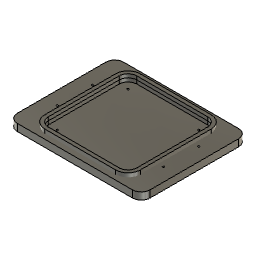
actu_board v5 (Autodesk Fusion 360 design; units mm, degrees)
Autodesk Fusion 360 part; units mm, degrees
sketch "스케치1" plane through (0, 0, 0) normal (0, 0, 1) x (1, 0, 0)
  line L0 (0, 100) -> (150, 100)
  line L1 (150, 100) -> (150, 0)
  line L2 (150, 0) -> (0, 0)
  line L3 (0, 0) -> (0, 100)
  dimension "d1" = 150
  dimension "d2" = 100
  constraint horizontal L0
  constraint vertical L1
  constraint horizontal L2
  constraint vertical L3
  constraint coincident L2.end L3.start
  measures "d1" distance of L0.start L0.end
  measures "d2" distance of L0.end L1.end
extrude "돌출1" add sketch "스케치1" along normal blind 8 makes body 1
sketch "스케치2" plane through (0, 0, 8) normal (0, 0, 1) x (-1, 0, 0)
  line L0 (0, 0) -> (-150, 0)
  line L1 (-150, 0) -> (-150, -100)
  line L2 (-150, -100) -> (0, -100)
  line L3 (0, -100) -> (0, 0)
  circle A0 centre (-15, -70) radius 1.25
  circle A1 centre (-135, -70) radius 1.25
  circle A2 centre (-35, -10) radius 1.25
  circle A3 centre (-115, -10) radius 1.25
  circle A4 centre (-15, -30) radius 1.25
  circle A5 centre (-35, -90) radius 1.25
  circle A6 centre (-135, -30) radius 1.25
  circle A7 centre (-115, -90) radius 1.25
  line L4 (0, 0) -> (0, -100)
  line L5 (-15, -100) -> (-15, 0) construction
  line L6 (-135, -100) -> (-135, 0) construction
  line L7 (-150, -100) -> (-150, 0)
  line L8 (0, -30) -> (-150, -30) construction
  line L9 (0, -70) -> (-150, -70) construction
  line L10 (-150, 0) -> (0, 0)
  line L11 (0, -100) -> (-150, -100)
  line L12 (-35, -100) -> (-35, 0) construction
  line L13 (-115, -100) -> (-115, 0) construction
  line L14 (0, -90) -> (-150, -90) construction
  line L15 (0, -10) -> (-150, -10) construction
  dimension "d9" = 2.5
  dimension "d11" = 15
  dimension "d12" = 15
  dimension "d13" = 30
  dimension "d14" = 30
  dimension "d15" = 35
  dimension "d16" = 35
  dimension "d17" = 10
  dimension "d18" = 10
  constraint equal A1 A6
  constraint equal A3 A7
  constraint equal A0 A1
  constraint equal A0 A4
  constraint equal A4 A5
  constraint equal A2 A5
  constraint equal A2 A3
  constraint coincident L2 L5.start
  constraint coincident L0 L5.end
  constraint perpendicular L0 L5
  constraint coincident L2 L6.start
  constraint coincident L0 L6.end
  constraint perpendicular L0 L6
  constraint coincident A0.centre L5
  constraint coincident A1.centre L6
  constraint coincident A4.centre L5
  constraint coincident A6.centre L6
  constraint coincident L4 L8.start
  constraint coincident L7 L8.end
  constraint perpendicular L7 L8
  constraint coincident L4 L9.start
  constraint coincident L7 L9.end
  constraint perpendicular L7 L9
  constraint coincident A4.centre L8
  constraint coincident A6.centre L8
  constraint coincident L11 L12.start
  constraint perpendicular L8 L12
  constraint coincident L11 L13.start
  constraint coincident L10 L13.end
  constraint perpendicular L10 L13
  constraint coincident L4 L14.start
  constraint coincident L7 L14.end
  constraint perpendicular L7 L14
  constraint coincident L4 L15.start
  constraint coincident L7 L15.end
  constraint perpendicular L7 L15
  constraint coincident A5.centre L12
  constraint coincident A5.centre L14
  constraint coincident A7.centre L13
  constraint coincident A7.centre L14
  constraint coincident A2.centre L12
  constraint coincident A3.centre L15
  constraint coincident A3.centre L13
  constraint coincident A2.centre L15
  measures "d9" diameter of A0
  measures "d11" distance of L4 L5
  measures "d12" distance of L6 L7
  measures "d13" distance of L8 L10
  measures "d14" distance of L9 L11
  measures "d15" distance of L4 L12
  measures "d16" distance of L7 L13
  measures "d17" distance of L11 L14
  measures "d18" distance of L10 L15
extrude "돌출3" cut sketch "스케치2" against normal blind 9 contours A0 | A1 | A2 | A3 | A4 | A5 | A6 | A7 bodies 1
thread "스레드1" "ISO Metric profile 2.5 M2.5x0.45 6H" major diameter 2.58 minor diameter 2.0755 pitch 0.45 angle 60 resizes the face on face at (33.7887, 89.6916, 2.6667) on bodies 1
thread "스레드2" "ISO Metric profile 2.5 M2.5x0.45 6H" major diameter 2.58 minor diameter 2.0755 pitch 0.45 angle 60 resizes the face on face at (13.7887, 69.6916, 2.6667) on bodies 1
thread "스레드3" "ISO Metric profile 2.5 M2.5x0.45 6H" major diameter 2.58 minor diameter 2.0755 pitch 0.45 angle 60 resizes the face on face at (13.7562, 30.1245, 2.6667) on bodies 1
thread "스레드4" "ISO Metric profile 2.5 M2.5x0.45 6H" major diameter 2.58 minor diameter 2.0755 pitch 0.45 angle 60 resizes the face on face at (33.7562, 10.1245, 2.6667) on bodies 1
thread "스레드5" "ISO Metric profile 2.5 M2.5x0.45 6H" major diameter 2.58 minor diameter 2.0755 pitch 0.45 angle 60 resizes the face on face at (114.6019, 8.8151, 2.6667) on bodies 1
thread "스레드6" "ISO Metric profile 2.5 M2.5x0.45 6H" major diameter 2.58 minor diameter 2.0755 pitch 0.45 angle 60 resizes the face on face at (134.7829, 28.769, 5.3333) on bodies 1
thread "스레드7" "ISO Metric profile 2.5 M2.5x0.45 6H" major diameter 2.58 minor diameter 2.0755 pitch 0.45 angle 60 resizes the face on face at (134.7829, 68.769, 5.3333) on bodies 1
thread "스레드8" "ISO Metric profile 2.5 M2.5x0.45 6H" major diameter 2.58 minor diameter 2.0755 pitch 0.45 angle 60 resizes the face on face at (114.6019, 88.8151, 2.6667) on bodies 1
extrude "돌출4" add 1 faces at (50, 100, 5.3333) along direction (0, 1, 0) blind 10 on bodies 1 bodies 1
extrude "돌출5" add 1 faces at (100, 0, 5.3333) along direction (0, -1, 0) blind 10 on bodies 1 bodies 1
sketch "스케치3" plane through (0, 0, 8) normal (0, 0, 1) x (-1, 0, 0)
  circle A0 centre (-135, -70) radius 1.0377
  circle A1 centre (-135, -30) radius 1.0377
  circle A2 centre (-35, -10) radius 1.0377
  circle A3 centre (-35, -90) radius 1.0377
  circle A4 centre (-15, -70) radius 1.0377
  circle A5 centre (-15, -30) radius 1.0377
  circle A6 centre (-115, -10) radius 1.0377
  circle A7 centre (-115, -90) radius 1.0377
  line L0 (-150, 10) -> (-150, -110)
  line L1 (-150, -110) -> (0, -110)
  line L2 (0, -110) -> (0, 10)
  line L3 (0, 10) -> (-150, 10)
  line L4 (-35, -100) -> (-115, -100)
  line L5 (-125, -90) -> (-125, -10)
  line L6 (-115, 0) -> (-35, 0)
  line L7 (-25, -10) -> (-25, -90)
  arc A8 (-35, -100) -> (-25, -90) centre (-35, -90) ccw
  arc A9 (-125, -90) -> (-115, -100) centre (-115, -90) ccw
  arc A10 (-115, 0) -> (-125, -10) centre (-115, -10) ccw
  arc A11 (-25, -10) -> (-35, 0) centre (-35, -10) ccw
  dimension "d27" = 10
  dimension "d28" = 10
  constraint horizontal L4
  constraint vertical L5
  constraint horizontal L6
  constraint vertical L7
  constraint tangent L4 A8
  constraint tangent L7 A8
  constraint tangent L4 A9
  constraint tangent L5 A9
  constraint tangent L5 A10
  constraint tangent L6 A10
  constraint equal A9 A10
  constraint tangent L6 A11
  constraint tangent L7 A11
  constraint equal A9 A11
  measures "d27" radius of A8
  measures "d28" radius of A9
extrude "돌출6" cut sketch "스케치3" against normal blind 4 contours L4 L5 L6 L7 A8 A9 A10 A11 bodies 1
sketch "스케치5" plane through (0, 0, 4) normal (0, 0, 1) x (-1, 0, 0)
  circle A0 centre (-115, -90) radius 1.0377
  circle A1 centre (-35, -90) radius 1.0377
  circle A2 centre (-35, -10) radius 1.0377
  circle A3 centre (-115, -10) radius 1.0377
  arc A4 (-35, -100) -> (-25, -90) centre (-35, -90) ccw
  line L0 (-25, -90) -> (-25, -10)
  arc A5 (-25, -10) -> (-35, 0) centre (-35, -10) ccw
  line L1 (-35, 0) -> (-115, 0)
  arc A6 (-115, 0) -> (-125, -10) centre (-115, -10) ccw
  line L2 (-125, -10) -> (-125, -90)
  arc A7 (-125, -90) -> (-115, -100) centre (-115, -90) ccw
  line L3 (-115, -100) -> (-35, -100)
  line L4 (-35, 4) -> (-115, 4)
  arc A8 (-115, 4) -> (-129, -10) centre (-115, -10) ccw
  line L5 (-129, -10) -> (-129, -90)
  arc A9 (-129, -90) -> (-115, -104) centre (-115, -90) ccw
  line L6 (-115, -104) -> (-35, -104)
  arc A10 (-35, -104) -> (-21, -90) centre (-35, -90) ccw
  line L7 (-21, -90) -> (-21, -10)
  arc A11 (-21, -10) -> (-35, 4) centre (-35, -10) ccw
  dimension "d34" = 4
extrude "돌출7" add sketch "스케치5" along normal blind 8 separate body contours L4 A8 L5 A9 L6 A10 L7 A11 makes body 2
fillet "모깎기1" radius 10 4 edges at (0, -10, 4) (150, -10, 4) (150, 110, 4) (0, 110, 4) on bodies 1
extrude "돌출2" [suppressed]
